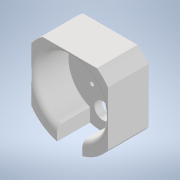
# Autodesk Inventor part: engine_cup
Saved by Autodesk Inventor 2020.1 (Build 241239000, 239)
## iProperties
Created: 2022-02-13
Part Number: engine_cup
Material: Generic
Document SubType Name: Modeling
Designer: OEM
Density: 1 g/cm^3
Appearance: Default
Author: OEM
Autodesk Inventor part; units mm, degrees
ref_plane "YZ Plane" through (0, 0, 0) normal (1, 0, 0) x (0, 1, 0)
ref_plane "XZ Plane" through (0, 0, 0) normal (0, 1, 0) x (-1, 0, 0)
ref_plane "XY Plane" through (0, 0, 0) normal (0, 0, 1) x (1, 0, 0)
sketch "Sketch1" plane through (0, 0, 0) normal (0, 0, 1) x (1, 0, 0)
  circle A0 centre (0, 0) radius 18.5 construction
  line L0 (0, 0) -> (17.9681, 0) construction
  line L1 (0, 0) -> (18.5, 0) construction
  line L2 (13.0815, -13.0815) -> (-13.0815, 13.0815) construction
  line L3 (0, 29) -> (0, -41) construction
  line L4 (-75, 0) -> (78, 0) construction
  line L5 (-13.0815, -13.0815) -> (13.0815, 13.0815) construction
  line L6 (-13.0815, 13.0815) -> (13.0815, 13.0815) construction
  line L7 (13.0815, -13.0815) -> (13.0815, 13.0815) construction
  line L8 (-13.0815, -13.0815) -> (-13.0815, 13.0815) construction
  circle A1 centre (-4.2426, 4.2426) radius 0.75
  circle A2 centre (4.2426, 4.2426) radius 0.75
  circle A3 centre (-4.2426, -4.2426) radius 0.75
  circle A4 centre (4.2426, -4.2426) radius 0.75
  circle A5 centre (0, 0) radius 13.5
  line L9 (10.7144, 15.0815) -> (-10.7144, 15.0815)
  line L10 (-15.0815, 10.7144) -> (-15.0815, -10.7144)
  line L11 (15.0815, 10.7144) -> (15.0815, -10.7144)
  arc A6 (-10.7144, 15.0815) -> (-15.0815, 10.7144) centre (0, 0) ccw
  arc A7 (15.0815, 10.7144) -> (10.7144, 15.0815) centre (0, 0) ccw
  line L12 (-5, -12.5399) -> (-5, -17.8115)
  line L13 (5, -12.5399) -> (5, -17.8115)
  arc A8 (-15.0815, -10.7144) -> (-5, -17.8115) centre (0, 0) ccw
  arc A9 (5, -17.8115) -> (15.0815, -10.7144) centre (0, 0) ccw
  arc A10 (-5, -17.8115) -> (5, -17.8115) centre (0, 0) ccw
  circle A11 centre (0, -11.25) radius 3.25
  circle A12 centre (0, 0) radius 6 construction
  point P0 (-2.5574, -13.2556)
  point P1 (2.5574, -13.2556)
  dimension "d0" = 37
  dimension "d7" = 27
  dimension "d27" = 12
  dimension "d3" = 45
  dimension "d4" = 1.5
  dimension "d9" = 2
  dimension "d10" = 2
  dimension "d11" = 5
  dimension "d22" = 6.5
  dimension "d25" = 11.25
  dimension "d26" = 18.5
  constraints: 28 end point, 10 centre point, 10 point on circle, 9 symmetric about line, 6 coincident, 5 horizontal, 2 perpendicular, 2 point on line, 2 vertical, 1 midpoint, 20 other
  measures "d3" angle of L0 L2
  measures "d4" diameter of A1
  measures "d9" distance between parallel lines of L6 L9
  measures "d10" distance between parallel lines of L10 L8
  measures "d11" distance between parallel lines of L12 L3
  measures "d22" diameter of A11
  measures "d25" distance from line of L4 A11.centre
  measures "d26" distance edge to line of A10 L4
extrude "Extrusion1" add sketch "Sketch1" along normal blind 3 contours A5 A11 | A5 A11 L13 A10 L12 | A11 A5 | A5 A11
extrude "Extrusion2" add sketch "Sketch1" along normal blind 16 contours A5 L12 A8 L10 A6 L9 A7 L11 A9 L13
fillet "Fillet2" radius 1 4 edges at (3.4926, 4.2426, 0) (3.4926, -4.2426, 0) (-4.9926, -4.2426, 0) (-4.9926, 4.2426, 0)
extrude "Extrusion3" cut sketch "Sketch1" along normal blind 16 contours A11 A5 | A5 A11 picked at (-0.1023, -11.6534) picked at (0, -13.8152)
fillet "Fillet3" radius 2 1 edges at (0, 13.5, 16)
body "Solid1"
